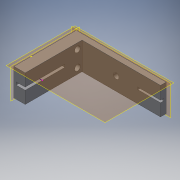
# Autodesk Inventor part: Gundaufbau
Saved by Autodesk Inventor 2017 (Build 210142000, 142)
## iProperties
Created: 2018-04-19
Part Number: Gundaufbau
Material: Allgemein
Document SubType Name: Modeling
Designer: pgmadmin
Density: 1 g/cm^3
Appearance: Vorgabe
Author: pgmadmin
Autodesk Inventor part; units mm, degrees
sketch "Skizze1" plane through (0, 0, 0) normal (0, 0, 1) x (1, 0, 0)
  line L0 (-15.8, 0) -> (94.8, 0) projected
  line L1 (0, -28.8) -> (0, 4.8) projected
  line L2 (0, 0) -> (79, 0)
  line L3 (79, 0) -> (79, -24)
  line L4 (79, -24) -> (0, -24)
  line L5 (0, -24) -> (0, 0)
  dimension "d0" = 79
  dimension "d1" = 24
  constraints: 8 end point, 2 parallel, 1 horizontal, 1 perpendicular
  measures "d0" distance of L3.end L4.end
  measures "d1" distance of L2.end L3.end
extrude "Extrusion1" add sketch "Skizze1" along normal blind 5
sketch "Skizze2" plane through (0, 0, 5) normal (0, 0, 1) x (1, 0, 0)
  line L0 (0, -24) -> (79, -24) projected
  line L1 (0, 0) -> (10, 0)
  line L2 (10, 0) -> (10, -24)
  line L3 (10, -24) -> (0, -24)
  line L4 (0, -24) -> (0, 0)
  dimension "d4" = 10
  constraints: 8 end point, 2 parallel, 1 horizontal, 1 perpendicular, 1 point on line
  measures "d4" distance between parallel lines of L4 L2
extrude "Extrusion2" add sketch "Skizze2" along normal blind 35
sketch "Skizze3" plane through (79, -24, 0) normal (1, 0, 0) x (0, 0, -1)
  line L0 (-5, 0) -> (-5, 24) projected
  line L1 (-5, 10.75) -> (-2, 10.75)
  line L2 (-2, 10.75) -> (-2, 12.75)
  line L3 (-2, 12.75) -> (-5, 12.75)
  line L4 (-5, 12.75) -> (-5, 10.75)
  line L5 (0, 24) -> (-5, 24) projected
  dimension "d7" = 3
  dimension "d8" = 2
  dimension "d9" = 11.25
  constraints: 8 end point, 2 parallel, 1 horizontal, 1 perpendicular, 1 point on line
  measures "d7" distance between parallel lines of L2 L0
  measures "d8" distance between parallel lines of L3 L1
  measures "d9" distance between parallel lines of L5 L3
extrude "Extrusion3" cut sketch "Skizze3" against normal blind 20
hole "Bohrung1" at (40, -12.25, 5) direction (0, 0, -1) diameter 5 end through all
sketch "Skizze5" plane through (0, -24, 0) normal (-1, 0, 0) x (0, 0, 1)
  line L0 (5, 24) -> (40, 24) projected
  line L1 (9, 24) -> (9, -0.204)
  line L2 (0, 0) -> (0, 24) projected
  circle A0 centre (9, 19) radius 2.55
  circle A1 centre (9, 5) radius 2.55
  line L3 (0, 0) -> (40, 0) projected
  dimension "d26" = 9
  dimension "d27" = 5.1
  dimension "d28" = 5.1
  dimension "d29" = 5
  dimension "d30" = 5
  constraints: 3 point on line, 2 centre point, 2 end point, 1 vertical
  measures "d26" distance between parallel lines of L1 L2
  measures "d27" diameter of A0
  measures "d28" diameter of A1
  measures "d29" distance from line of L3 A1.centre
  measures "d30" distance from line of A0.centre L0
extrude "Extrusion5" cut sketch "Skizze5" against normal blind 30
sketch "Skizze6" plane through (0, 0, 40) normal (0, 0, 1) x (1, 0, 0)
  line L0 (79, -24) -> (0, -24) projected
  line L1 (0, 0) -> (0, -24)
  line L2 (0, -24) -> (10, -24)
  line L3 (10, -24) -> (10, -13.4534)
  line L4 (10, 0) -> (10, -24) projected
  line L5 (10, -13.25) -> (2, -13.25) projected
  line L6 (2, -11.25) -> (10, -11.25) projected
  line L7 (2, -13.25) -> (2, -11.25)
  line L8 (2, -11.25) -> (10, -11.25)
  line L9 (10, -11.25) -> (10, 0)
  line L10 (0, 0) -> (79, 0) projected
  line L11 (0, -24) -> (0, 0) projected
  line L12 (0, 0) -> (0, -24)
  dimension "d33" = 10
  constraints: 14 end point, 4 point on line, 2 perpendicular, 2 vertical
  measures "d33" distance of L0.end L2.end
sketch "Skizze7" plane through (0, 0, 40) normal (0, 0, 1) x (1, 0, 0)
  line L0 (10, -13.25) -> (2, -13.25) projected
  line L1 (2, -13.25) -> (10, -13.25)
  point P0 (0, 0)
  constraints: 2 end point, 1 collinear
extrude "Extrusion6" add sketch "Skizze6" along normal blind 15 contours L0 L1 L10 L4 L6 L7 L5 L3
sketch "Skizze8" plane through (0, 0, 55) normal (0, 0, 1) x (1, 0, 0)
  line L0 (10, -11.25) -> (2, -11.25) projected
  line L1 (2, -13.25) -> (10, -13.25) projected
  line L2 (2, -11.25) -> (2, -13.25)
  line L3 (2, -13.25) -> (10, -13.25)
  line L4 (10, -13.25) -> (10, -11.25)
  line L5 (10, 0) -> (10, -24) projected
  line L6 (2, -11.25) -> (10, -11.25)
  point P0 (0, 0)
  constraints: 8 end point, 1 collinear, 1 perpendicular, 1 point on line, 1 vertical
extrude "Extrusion7" add sketch "Skizze8" against normal blind 35
sketch "Skizze9" plane through (0, 0, 0) normal (0, 1, 0) x (-1, 0, 0)
  point P0 (0, 0)
sketch "Skizze10" plane through (0, 0, 55) normal (0, 0, 1) x (1, 0, 0)
  line L0 (10, 0) -> (10, -24) projected
  line L1 (10, -13.25) -> (2, -13.25)
  line L2 (2, -13.25) -> (2, -10.75)
  line L3 (2, -10.75) -> (10, -10.75)
  line L4 (10, -10.75) -> (10, -13.25)
  line L5 (10, 0) -> (0, 0) projected
  line L6 (0, -24) -> (10, -24) projected
  dimension "d38" = 8
  dimension "d39" = 10.75
  dimension "d40" = 10.75
  constraints: 8 end point, 2 parallel, 1 horizontal, 1 perpendicular, 1 point on line
  measures "d38" distance between parallel lines of L2 L0
  measures "d39" distance between parallel lines of L5 L3
  measures "d40" distance between parallel lines of L1 L6
extrude "Extrusion8" cut sketch "Skizze10" against normal blind 35
